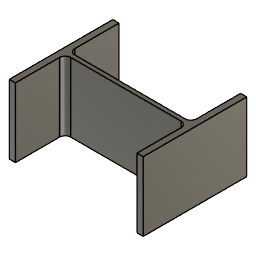
H-194×150×6×9 (Autodesk Fusion 360 design; units mm, degrees)
Autodesk Fusion 360 part; units mm, degrees
sketch "スケッチ1" plane through (0, 0, 0) normal (0, 0, 1) x (1, 0, 0)
  line L0 (0, 75) -> (0, -75)
  line L1 (9, -75) -> (9, -11)
  line L2 (0, -75) -> (9, -75)
  line L3 (9, 11) -> (9, 75)
  line L4 (9, 75) -> (0, 75)
  line L5 (194, -75) -> (194, 75)
  line L6 (185, -11) -> (185, -75)
  line L7 (185, -75) -> (194, -75)
  line L8 (177, 3) -> (17, 3)
  line L9 (17, -3) -> (177, -3)
  line L10 (185, 75) -> (185, 11)
  line L11 (194, 75) -> (185, 75)
  arc A0 (17, -3) -> (9, -11) centre (17, -11) ccw
  arc A1 (9, 11) -> (17, 3) centre (17, 11) ccw
  arc A2 (177, 3) -> (185, 11) centre (177, 11) ccw
  arc A3 (185, -11) -> (177, -3) centre (177, -11) ccw
extrude "押し出し1" add sketch "スケッチ1" along normal blind 100
